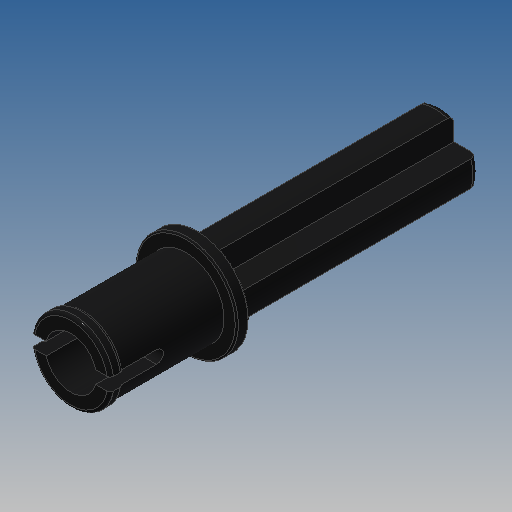
# Autodesk Inventor part: 18651-Black
Saved by Autodesk Inventor 2022.2 (Build 262287000, 287)
## iProperties
Created: 2014-06-03
Part Number: 18651-Black
Material: ABS Plastic
Document SubType Name: Modeling
Designer: D. Kohfeld
Appearance: Black
Density: 1.06 g/cm^3
Mass: 0.300013 g
Surface Area: 5.32149 cm^2
Volume: 0.283031 cm^3
Author: D. Kohfeld
Autodesk Inventor part; units mm, degrees
ref_plane "YZ Plane" through (0, 0, 0) normal (1, 0, 0) x (0, 1, 0)
ref_plane "XZ Plane" through (0, 0, 0) normal (0, 1, 0) x (-1, 0, 0)
ref_plane "XY Plane" through (0, 0, 0) normal (0, 0, 1) x (1, 0, 0)
sketch "Sketch1" plane through (0, 0, 0) normal (0, 1, 0) x (-1, 0, 0)
  line L0 (2.4, 7.2) -> (2.4, 0.8)
  line L1 (3.2, 0.8) -> (2.4, 0.8)
  line L2 (3.2, 0.8) -> (3.2, 0)
  line L3 (0, 0) -> (3.2, 0)
  line L4 (2.5, 8) -> (2.5, 7.2)
  line L5 (2.5, 8) -> (1.6, 8)
  line L6 (0, -1.6) -> (0, 9.6) projected
  line L7 (2.4, 7.2) -> (2.5, 7.2)
  line L8 (3.72, 0) -> (-0.62, 0) projected
  line L9 (0, 0) -> (0, 0.8)
  line L10 (0, 0.8) -> (1.6, 0.8)
  line L11 (1.6, 8) -> (1.6, 0.8)
  dimension "d1" = 4.8
  dimension "d2" = 5
  dimension "d7" = 0.8
  dimension "d8" = 6.4
  dimension "d9" = 0.8
  dimension "d40" = 3.2
  dimension "d44" = 0
  dimension "d46" = 8
  constraints: 20 end point, 2 perpendicular, 2 point on line, 1 horizontal, 1 horizontal alignment, 1 parallel
  measures "d1" diameter of L0 L6
  measures "d2" diameter of L4 L6
  measures "d7" distance from line of L4.end L5
  measures "d8" diameter of L2 L6
  measures "d9" distance between parallel lines of L1 L8
  measures "d40" diameter of L11 L6
  measures "d44" distance between parallel lines of L3 L8
  measures "d46" distance between parallel lines of L5 L8
revolve "Revolution1" add sketch "Sketch1" angle 360 about axis through (0, 0, -10) along (0, 0, 1)
fillet "Fillet1" radius 0.2 2 edges at (2.5, 0, 8) (2.5, 0, 7.2)
fillet "Fillet1" radius 0.1 2 edges at (3.2, 0, 0.8) (3.2, 0, 0)
sketch "Sketch2" plane through (0, 0, 0) normal (1, 0, 0) x (0, 1, 0)
  line L0 (-1.6, 8) -> (1.6, 8) projected
  line L1 (-0.4, 8) -> (0.4, 8)
  line L2 (0.4, 8) -> (0.4, 5)
  line L3 (-0.4, 5) -> (-0.4, 8)
  arc A0 (-0.4, 5) -> (0.4, 5) centre (0, 5) ccw
  point P0 (0, 0)
  point P1 (0, 8)
  dimension "d34" = 3.4
  dimension "d41" = 0.8
  constraints: 6 end point, 2 midpoint, 2 point on circle, 2 tangent, 1 centre point, 1 horizontal, 1 parallel, 1 perpendicular, 1 point on line
  measures "d41" distance between parallel lines of L2 L3
extrude "Extrusion2" cut sketch "Sketch2" along normal through all both and the other way through all
sketch "Sketch3" plane through (0, 0, 0) normal (0, 0, -1) x (-1, 0, 0)
  circle A0 centre (0, 0) radius 3.1 projected
  circle A1 centre (0, 0) radius 2.4 construction
  line L0 (-0.8, 2.2627) -> (-0.8, 0.8)
  line L1 (-0.8, 0.8) -> (-2.2627, 0.8)
  line L2 (-2.2627, -0.8) -> (-0.8, -0.8)
  line L3 (-0.8, -0.8) -> (-0.8, -2.2627)
  line L4 (0.8, -2.2627) -> (0.8, -0.8)
  line L5 (0.8, -0.8) -> (2.2627, -0.8)
  line L6 (2.2627, 0.8) -> (0.8, 0.8)
  line L7 (0.8, 0.8) -> (0.8, 2.2627)
  arc A2 (0.8, 2.2627) -> (-0.8, 2.2627) centre (0, 0) ccw
  arc A3 (-2.2627, 0.8) -> (-2.2627, -0.8) centre (0, 0) ccw
  arc A4 (-0.8, -2.2627) -> (0.8, -2.2627) centre (0, 0) ccw
  arc A5 (2.2627, -0.8) -> (2.2627, 0.8) centre (0, 0) ccw
  dimension "d35" = 4.8
  dimension "d36" = 1.6
  constraints: 16 end point, 8 point on circle, 7 equal length, 4 centre point, 4 perpendicular, 3 parallel, 1 coincident, 1 vertical, 14 other
  measures "d36" distance between parallel lines of L0 L7
extrude "Extrusion3" add sketch "Sketch3" along normal blind 15.2 contours A2 L7 L6 A5 L5 L4 A4 L3 L2 A3 L1 L0
fillet "Fillet2" radius 0.4 4 edges at (0, 2.4, -15.2) (2.4, 0, -15.2) (0, -2.4, -15.2) (-2.4, 0, -15.2)
equation "\"d1\" = tpd"
equation "\"d2\" = tpcd"
equation "\"d7\" = d9"
equation "\"d8\" = tsd"
equation "\"d9\" = tsl"
equation "\"d40\" = rd"
equation "\"d46\" = lu"
equation "\"d27\" = pinf"
equation "\"d28\" = lf"
equation "\"d34\" = tpnl"
equation "\"d41\" = tpnw"
equation "\"d35\" = kd"
equation "\"d36\" = axlet"
equation "\"d37\" = 2 * lu - tsl"
equation "\"d39\" = tf"
equation "\"tpd\" = 4.8"
equation "\"tpcd\" = 5"
equation "\"tsd\" = 6.4"
equation "\"tsl\" = 0.8"
equation "\"rd\" = 3.2"
equation "\"lu\" = 8"
equation "\"pinf\" = 0.2"
equation "\"lf\" = 0.1"
equation "\"tpnl\" = 3.4"
equation "\"tpnw\" = 0.8"
equation "\"kd\" = 4.8"
equation "\"axlet\" = 1.6"
equation "\"tf\" = 0.4"
body "Solid2"
